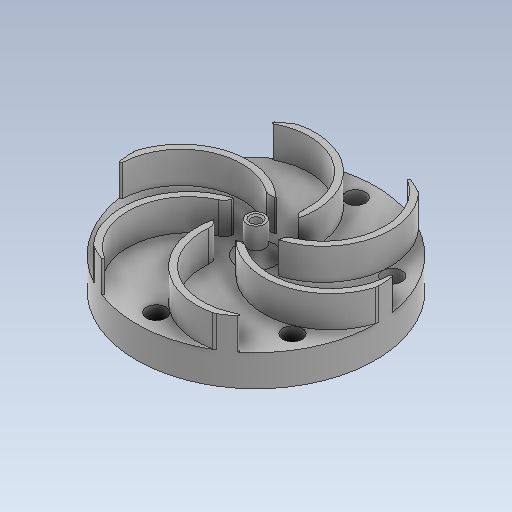
# Autodesk Inventor part: impeller_right
Saved by Autodesk Inventor 2020.1 (Build 241239000, 239)
## iProperties
Created: 2019-10-27
Part Number: impeller_right
Material: PMMA Plastic
Document SubType Name: Modeling
Designer: agmle
Density: 1.188 g/cm^3
Appearance: Smooth - Medium Gray
Mass: 58.5336 g
Surface Area: 183.876 cm^2
Volume: 49.2707 cm^3
Author: agmle
Autodesk Inventor part; units mm, degrees
ref_plane "YZ Plane" through (0, 0, 0) normal (1, 0, 0) x (0, 1, 0)
ref_plane "XZ Plane" through (0, 0, 0) normal (0, 1, 0) x (-1, 0, 0)
ref_plane "XY Plane" through (0, 0, 0) normal (0, 0, 1) x (1, 0, 0)
sketch "Sketch1" plane through (0, 0, 0) normal (0, 1, 0) x (-1, 0, 0)
  circle A0 centre (0, 0) radius 38.1
  dimension "d0" = 76.2
  constraints: 1 centre point, 1 coincident
  measures "d0" diameter of A0
extrude "Drive Platen" add sketch "Sketch1" along normal blind 10
sketch "Sketch2" plane through (0, 10, 0) normal (0, 1, 0) x (1, 0, 0)
  circle A0 centre (0, 0) radius 2.8575
  dimension "d3" = 5.715
  constraints: 1 centre point, 1 coincident
  measures "d3" diameter of A0
extrude "Shaft Housing" add sketch "Sketch2" along normal blind 10 and the other way blind 10.5
sketch "Sketch3" plane through (0, 20, 0) normal (0, 1, 0) x (1, 0, 0)
  point P0 (0, 0)
  point P1 (0, 0)
  constraints: 1 coincident
hole "Shaft Bore" at (0, 20, 0) direction (0, -1, 0) diameter 3.175 end through all
sketch "Sketch4" plane through (0, 10, 0) normal (0, 1, 0) x (1, 0, 0)
  circle A0 centre (0, -31.825) radius 3.1 construction
  circle A1 centre (0, 0) radius 1.5875 construction
  line L0 (0, -31.825) -> (0, 0) construction
  circle A2 centre (27.5613, -15.9125) radius 3.1 construction
  circle A3 centre (27.5613, 15.9125) radius 3.1 construction
  circle A4 centre (0, 31.825) radius 3.1 construction
  circle A5 centre (-27.5613, 15.9125) radius 3.1 construction
  circle A6 centre (-27.5613, -15.9125) radius 3.1 construction
  line L1 (-12.6599, -34.925) -> (7.5493, -34.925) construction
  line L2 (-8.1083, -38.1) -> (6.3962, -38.1) construction
  circle A7 centre (0, 0) radius 38.1 construction
  dimension "d13" = 6.2
  dimension "d16" = 360
  dimension "d18" = 3.175
  constraints: 6 centre point, 6 coincident, 6 end point, 2 horizontal, 2 tangent, 1 vertical, 19 other
  measures "d13" diameter of A0
  measures "d18" distance between parallel lines of L2 L1
hole "Magnets" at (0, 10, 31.825) at (27.5613, 10, 15.9125) at (27.5613, 10, -15.9125) at (0, 10, -31.825) at (-27.5613, 10, -15.9125) at (-27.5613, 10, 15.9125) direction (0, -1, 0) diameter 6.2 depth 10
sketch "Sketch5" plane through (0, 10, 0) normal (0, 1, 0) x (1, 0, 0)
  circle A0 centre (0, 0) radius 38.1 projected
  arc A1 (2.7125, -9.1306) -> (37.9392, 0.0373) centre (17.4531, 6.4915) ccw
  circle A2 centre (0, 0) radius 2.8575 construction
  circle A3 centre (0, 0) radius 9.525 construction
  arc A4 (6.1406, -9.3656) -> (36.9177, 5.7492) centre (17.4531, 6.4915) ccw
  circle A5 centre (0, 0) radius 38.1 construction
  arc A6 (38.0846, 1.0815) -> (37.6572, 5.7916) centre (0, 0) ccw
  arc A7 (2.7125, -9.1306) -> (3.2195, -8.9637) centre (-0.0123, -0.0037) ccw
  arc A8 (6.1406, -9.3656) -> (3.2195, -8.9637) centre (4.2967, -11.9503) ccw
  arc A9 (37.9392, 0.0373) -> (38.0846, 1.0815) centre (34.9109, 0.9914) ccw
  arc A10 (37.6572, 5.7916) -> (36.9177, 5.7492) centre (37.2895, 5.735) ccw
  arc A11 (9.2636, -2.2162) -> (18.9373, 32.8749) centre (3.1047, 18.3606) ccw
  arc A12 (9.2636, -2.2162) -> (9.3725, -1.6937) centre (-0.003, -0.0125) ccw
  arc A13 (11.1812, 0.6351) -> (9.3725, -1.6937) centre (12.4976, -2.2541) ccw
  arc A14 (11.1812, 0.6351) -> (13.4799, 34.8463) centre (3.1047, 18.3606) ccw
  arc A15 (13.813, 35.5079) -> (13.4799, 34.8463) centre (13.6781, 35.1612) ccw
  arc A16 (18.1057, 33.523) -> (13.813, 35.5079) centre (0, 0) ccw
  arc A17 (18.9373, 32.8749) -> (18.1057, 33.523) centre (16.5969, 30.7294) ccw
  arc A18 (6.5511, 6.9144) -> (-19.0019, 32.8377) centre (-14.3484, 11.8691) ccw
  arc A19 (6.5511, 6.9144) -> (6.153, 7.27) centre (0.0093, -0.0088) ccw
  arc A20 (5.0406, 10.0007) -> (6.153, 7.27) centre (8.2009, 9.6962) ccw
  arc A21 (5.0406, 10.0007) -> (-23.4378, 29.0971) centre (-14.3484, 11.8691) ccw
  arc A22 (-23.8443, 29.7163) -> (-23.4378, 29.0971) centre (-23.6114, 29.4261) ccw
  arc A23 (-19.9789, 32.4415) -> (-23.8443, 29.7163) centre (0, 0) ccw
  arc A24 (-19.0019, 32.8377) -> (-19.9789, 32.4415) centre (-18.314, 29.7381) ccw
  arc A25 (-2.7125, 9.1306) -> (-37.9392, -0.0373) centre (-17.4531, -6.4915) ccw
  arc A26 (-2.7125, 9.1306) -> (-3.2195, 8.9637) centre (0.0123, 0.0037) ccw
  arc A27 (-6.1406, 9.3656) -> (-3.2195, 8.9637) centre (-4.2967, 11.9503) ccw
  arc A28 (-6.1406, 9.3656) -> (-36.9177, -5.7492) centre (-17.4531, -6.4915) ccw
  arc A29 (-37.6572, -5.7916) -> (-36.9177, -5.7492) centre (-37.2895, -5.735) ccw
  arc A30 (-38.0846, -1.0815) -> (-37.6572, -5.7916) centre (0, 0) ccw
  arc A31 (-37.9392, -0.0373) -> (-38.0846, -1.0815) centre (-34.9109, -0.9914) ccw
  arc A32 (-9.2636, 2.2162) -> (-18.9373, -32.8749) centre (-3.1047, -18.3606) ccw
  arc A33 (-9.2636, 2.2162) -> (-9.3725, 1.6937) centre (0.003, 0.0125) ccw
  arc A34 (-11.1812, -0.6351) -> (-9.3725, 1.6937) centre (-12.4976, 2.2541) ccw
  arc A35 (-11.1812, -0.6351) -> (-13.4799, -34.8463) centre (-3.1047, -18.3606) ccw
  arc A36 (-13.813, -35.5079) -> (-13.4799, -34.8463) centre (-13.6781, -35.1612) ccw
  arc A37 (-18.1057, -33.523) -> (-13.813, -35.5079) centre (0, 0) ccw
  arc A38 (-18.9373, -32.8749) -> (-18.1057, -33.523) centre (-16.5969, -30.7294) ccw
  arc A39 (-6.5511, -6.9144) -> (19.0019, -32.8377) centre (14.3484, -11.8691) ccw
  arc A40 (-6.5511, -6.9144) -> (-6.153, -7.27) centre (-0.0093, 0.0088) ccw
  arc A41 (-5.0406, -10.0007) -> (-6.153, -7.27) centre (-8.2009, -9.6962) ccw
  arc A42 (-5.0406, -10.0007) -> (23.4378, -29.0971) centre (14.3484, -11.8691) ccw
  arc A43 (23.8443, -29.7163) -> (23.4378, -29.0971) centre (23.6114, -29.4261) ccw
  arc A44 (19.9789, -32.4415) -> (23.8443, -29.7163) centre (0, 0) ccw
  arc A45 (19.0019, -32.8377) -> (19.9789, -32.4415) centre (18.314, -29.7381) ccw
  circle A46 centre (27.5613, -15.9125) radius 3.1 projected
  point P0 (18.1057, 33.523)
  point P1 (13.813, 35.5079)
  point P2 (-19.9789, 32.4415)
  point P3 (-23.8443, 29.7163)
  point P4 (-38.0846, -1.0815)
  point P5 (-37.6572, -5.7916)
  point P6 (-18.1057, -33.523)
  point P7 (-13.813, -35.5079)
  point P8 (19.9789, -32.4415)
  point P9 (23.8443, -29.7163)
  point P10 (38.0846, 1.0815)
  point P11 (37.6572, 5.7916)
  dimension "d27" = 19.05
  dimension "d28" = 2
  dimension "d29" = 3.175
  dimension "d30" = 0.3721
  dimension "d33" = 360
  constraints: 84 point on circle, 42 centre point, 9 tangent, 6 concentric, 1 coincident, 1 equal radius, 135 other
  measures "d28" radial gap between concentric circles of A1 A4
  measures "d29" radius of A8
  measures "d30" radius of A10
extrude "Vanes" add sketch "Sketch5" along normal blind 10 contours A9 A1 A7 A8 A4 A10 A0 | A0 A45 A39 A40 A41 A42 A43 | A17 A11 A12 A13 A14 A15 A0 | A0 A38 A32 A33 A34 A35 A36 | A24 A18 A19 A20 A21 A22 A0 | A0 A31 A25 A26 A27 A28 A29
fillet "Shaft strength" radius 3.175 1 edges at (-2.8575, 10, 0)
fillet "Offset strength" radius 0.5 1 edges at (-2.8575, 0, 0)
chamfer "Leadin" distance 0.5 angle 45 8 edges at (0, 20, -1.5875) (0, -0.5, -1.5875) (27.5613, 0, 12.8125) (0, 0, 28.725) (-27.5613, 0, 12.8125) (-27.5613, 0, -19.0125) (0, 0, -34.925) (27.5613, 0, -19.0125)
equation "\"d0\" = impeller_od"
equation "\"d1\" = 0.5 * impeller_height"
equation "\"d3\" = impeller_shaft_od"
equation "\"d4\" = 0.5 * impeller_height"
equation "\"d38\" = 0.5 * impeller_height + impeller_clearance"
equation "\"d6\" = impeller_shaft_id"
equation "\"d13\" = magnet_od + magnet_clearance"
equation "\"d19\" = magnet_od + magnet_clearance"
equation "\"d24\" = magnet_length"
equation "\"d27\" = impeller_intake_od"
equation "\"d28\" = impeller_vane_thick"
equation "\"d29\" = impeller_vane_inner_rad"
equation "\"d30\" = impeller_vane_outer_rad"
equation "\"d35\" = 0.5 * impeller_height"
equation "\"d43\" = impeller_shaft_support"
equation "\"d45\" = impeller_clearance"
equation "\"d47\" = 2 * magnet_clearance"
equation "\"hull_od\" = 219.075"
equation "\"hull_id\" = 201.7268"
equation "\"hull_wall\" = 8.6741"
equation "\"hull_length\" = 609.6"
equation "\"hull_spacing\" = 390.525"
equation "\"impeller_od\" = 76.2"
equation "\"impeller_clearance\" = 0.5"
equation "\"impeller_shaft_id\" = 3.175"
equation "\"impeller_shaft_od\" = 5.715"
equation "\"impeller_shaft_support\" = 3.175"
equation "\"impeller_intake_od\" = 19.05"
equation "\"impeller_vane_thick\" = 2"
equation "\"impeller_vane_inner_rad\" = 3.175"
equation "\"impeller_vane_outer_rad\" = 0.37206"
equation "\"magnet_od\" = 5.95"
equation "\"magnet_length\" = 10"
equation "\"magnet_clearance\" = 0.25"
equation "\"magnet_rad\" = 0.25"
equation "\"magnet_circle_offset\" = 3.175"
equation "\"motor_shaft_od\" = 12.7"
equation "\"motor_shaft_length\" = 31.75"
equation "\"motor_shaft_key\" = 3.048"
equation "\"impeller_height\" = 20"
body "Solid1"
